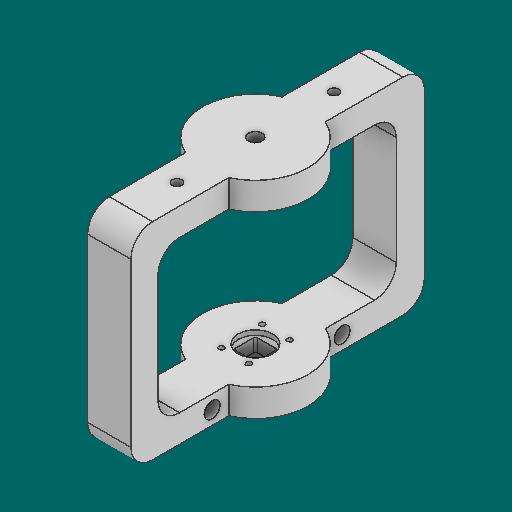
# Autodesk Inventor part: Linear_Odom
Saved by Autodesk Inventor 2025.2 (Build 292293000, 293)
## iProperties
Created: 2024-11-26
Part Number: Linear_Odom
Material: Generic
Document SubType Name: Modeling
Designer: AtuStem
Density: 1 g/cm^3
Appearance: Default
Author: AtuStem
Autodesk Inventor part; units mm, degrees
ref_plane "YZ Plane" through (0, 0, 0) normal (1, 0, 0) x (0, 1, 0)
ref_plane "XZ Plane" through (0, 0, 0) normal (0, 1, 0) x (-1, 0, 0)
ref_plane "XY Plane" through (0, 0, 0) normal (0, 0, 1) x (1, 0, 0)
sketch "Sketch1" plane through (0, 0, 0) normal (0, 1, 0) x (-1, 0, 0)
  line L0 (-6.75, -8.275) -> (-6.75, 8.275)
  line L1 (-6.75, -8.275) -> (6.75, -8.275)
  line L2 (6.75, -8.275) -> (6.75, 8.275)
  line L3 (6.75, 8.275) -> (-6.75, 8.275)
  circle A0 centre (4, 6) radius 0.8
  circle A1 centre (4, -6) radius 0.8
  circle A2 centre (-4, 6) radius 0.8
  circle A3 centre (-4, -6) radius 0.8
  line L4 (-5.98, -14.3) -> (-3.115, -23.927)
  arc A4 (-3.115, -23.927) -> (3.115, -23.927) centre (0, -23) ccw
  line L5 (3.115, -23.927) -> (5.98, -14.3)
  arc A5 (5.98, -14.3) -> (14.8963, -4.2836) centre (0, 0) ccw
  arc A6 (14.8963, 4.2836) -> (5.98, 14.3) centre (0, 0) ccw
  line L6 (5.98, 14.3) -> (3.115, 23.927)
  arc A7 (3.115, 23.927) -> (-3.115, 23.927) centre (0, 23) ccw
  line L7 (-3.115, 23.927) -> (-5.98, 14.3)
  circle A8 centre (0, -23.0125) radius 1.435
  circle A9 centre (0, 23.0125) radius 1.435
  circle A10 centre (0, 0) radius 15.5
  line L8 (0, 0) -> (0, 34.925)
  line L9 (0, 0) -> (0, -34.925)
  line L10 (0, -34.925) -> (0, -43.18)
  line L11 (0, 34.925) -> (0, 43.18)
  line L12 (0, -43.18) -> (-6.35, -43.18)
  line L13 (0, -43.18) -> (6.35, -43.18)
  line L14 (-6.35, -43.18) -> (6.35, -43.18)
  line L15 (6.35, -43.18) -> (6.35, -34.925)
  line L16 (6.35, -34.925) -> (-6.35, -34.925)
  line L17 (-6.35, -34.925) -> (-6.35, -43.18)
  line L18 (-6.35, 34.925) -> (6.35, 34.925)
  line L19 (6.35, 34.925) -> (6.35, 42.8439)
  line L20 (6.35, 42.8439) -> (-6.35, 42.8439)
  line L21 (-6.35, 42.8439) -> (-6.35, 34.925)
  line L22 (-6.35, -34.925) -> (-6.35, -14.1396)
  line L23 (-6.35, -14.1396) -> (-6.35, -13.0566)
  line L24 (-6.35, 14.1396) -> (-6.35, 34.925)
  line L25 (6.35, -34.925) -> (6.35, -14.1396)
  line L26 (6.35, 14.1396) -> (6.35, 34.925)
  point P0 (0, 0)
  point P1 (0, 0)
  point P2 (0, 0)
  point P3 (14.8963, -4.2836)
  point P4 (14.8963, 4.2836)
  dimension "d11" = 34.925
  dimension "d12" = 34.925
  dimension "d13" = 8.255
  dimension "d14" = 8.255
  dimension "d15" = 6.35
  dimension "d16" = 6.35
  constraints: 54 end point, 12 point on circle, 11 centre point, 7 vertical, 4 horizontal, 4 parallel, 4 perpendicular, 1 coincident, 1 point on line
  measures "d11" distance of L8.start L8.end
  measures "d12" distance of L8.start L9.end
  measures "d13" distance of L9.end L10.end
  measures "d14" distance of L8.end L11.end
  measures "d15" distance of L10.end L12.end
  measures "d16" distance of L10.end L13.end
extrude "Extrusion1" add sketch "Sketch1" along normal blind 8.001 contours L0 L3 L8 L9 L1 | L9 L8 L3 L2 L1
sketch "Sketch2" plane through (0, 8.001, 0) normal (0, 1, 0) x (1, 0, 0)
  circle A0 centre (0, 0) radius 5.08
  dimension "d4" = 10.16
  constraints: 1 centre point, 1 coincident
  measures "d4" diameter of A0
extrude "Extrusion2" cut sketch "Sketch2" against normal blind 1.397
sketch "Sketch3" plane through (0, 6.604, 0) normal (0, 1, 0) x (1, 0, 0)
  line L0 (-3.2283, 2.5775) -> (-3.2283, -2.5775)
  arc A0 (-3.2283, -2.5775) -> (-2.5775, -3.2283) centre (-2.5775, -2.5775) ccw
  line L1 (-2.5775, -3.2283) -> (2.5775, -3.2283)
  arc A1 (2.5775, -3.2283) -> (3.2283, -2.5775) centre (2.5775, -2.5775) ccw
  line L2 (3.2283, -2.5775) -> (3.2283, 2.5775)
  arc A2 (3.2283, 2.5775) -> (2.5775, 3.2283) centre (2.5775, 2.5775) ccw
  line L3 (2.5775, 3.2283) -> (-2.5775, 3.2283)
  arc A3 (-2.5775, 3.2283) -> (-3.2283, 2.5775) centre (-2.5775, 2.5775) ccw
  circle A4 centre (0, 0) radius 2.0828
  constraints: 8 end point, 8 point on circle, 5 centre point
extrude "Extrusion3" cut sketch "Sketch3" against normal blind 3.81 contours A3 L3 A2 L2 A1 L1 A0 L0 | A4
extrude "Extrusion4" add sketch "Sketch1" along normal up to surface (8.001 mm away) contours L1 L9 A10 L8 L3 L0 | L1 L2 L3 L8 A10 A6 A5 L9 | L9 A8 A4 L4 A10 | A10 L5 A4 L9 A8 | L8 A9 A7 L6 A10 | A10 L7 A7 L8 A9
extrude "Extrusion5" add sketch "Sketch1" along normal up to surface (8.001 mm away) contours L4 A4 L9 L16 L22 A10 | A5 L25 L16 L9 A4 L5 | L6 A7 L8 L18 L26 A6 | A10 L24 L18 L8 A7 L7
extrude "Extrusion6" add sketch "Sketch1" along normal up to surface (8.001 mm away) contours L16 L10 L12 L17 | L15 L13 L10 L16 | L18 L11 L20 L19 | L21 L20 L11 L18
sketch "Sketch5" plane through (0, 8.001, 0) normal (0, 1, 0) x (1, 0, 0)
  arc A0 (6.35, -14.1396) -> (6.35, 14.1396) centre (0, 0) ccw projected
  line L0 (6.35, 43.18) -> (6.35, 14.1396) projected
  line L1 (-6.35, 43.18) -> (6.35, 43.18) projected
  line L2 (-6.35, 14.1396) -> (-6.35, 43.18) projected
  arc A1 (-6.35, 14.1396) -> (-6.35, -14.1396) centre (0, 0) ccw projected
  line L3 (-6.35, -42.8439) -> (-6.35, -14.1396) projected
  line L4 (6.35, -42.8439) -> (-6.35, -42.8439) projected
  line L5 (6.35, -14.1396) -> (6.35, -42.8439) projected
  circle A2 centre (0, 23.0125) radius 1.435 projected
  circle A3 centre (0, -23.0125) radius 1.435 projected
  circle A4 centre (0, 0) radius 5.08 projected
  circle A5 centre (-4, -6) radius 0.8 projected
  circle A6 centre (-4, 6) radius 0.8 projected
  circle A7 centre (4, -6) radius 0.8 projected
  circle A8 centre (4, 6) radius 0.8 projected
  line L6 (-6.35, 34.925) -> (6.35, 34.925) projected
  line L7 (6.35, -34.925) -> (-6.35, -34.925) projected
extrude "Extrusion7" add sketch "Sketch5" along normal blind 44.45 contours L5 L4 L3 L7 | L6 L2 L1 L0
fillet "Fillet1" radius 6.35 2 edges at (0, 8.001, -34.925) (0, 8.001, 34.925)
sketch "Sketch6" plane through (0, 52.451, 0) normal (0, 1, 0) x (1, 0, 0)
  line L0 (-6.35, 34.925) -> (6.35, 34.925) projected
  line L1 (-6.35, 43.18) -> (-6.35, 34.925) projected
  line L2 (-6.35, 34.925) -> (6.35, 34.925) projected
  line L3 (6.35, 34.925) -> (6.35, 43.18) projected
  line L4 (6.35, 43.18) -> (-6.35, 43.18) projected
  line L5 (6.35, -42.8439) -> (6.35, -34.925) projected
  line L6 (6.35, -34.925) -> (-6.35, -34.925) projected
  line L7 (-6.35, -34.925) -> (-6.35, -42.8439) projected
  line L8 (-6.35, -42.8439) -> (6.35, -42.8439) projected
  point P0 (0, 0)
extrude "Extrusion8" add sketch "Sketch6" along normal blind 8.001
sketch "Sketch7" plane through (-6.35, 0, 42.8439) normal (0, 0, 1) x (1, 0, 0)
  line L0 (0, 0) -> (0, 60.452) projected
  line L1 (0, 0) -> (12.7, 0) projected
  line L2 (12.7, 0) -> (12.7, 60.452) projected
  line L3 (0, 60.452) -> (12.7, 60.452) projected
  line L4 (0, 60.452) -> (0, 52.451)
  line L5 (0, 52.451) -> (12.7, 52.451)
  point P0 (6.35, 0)
  dimension "d26" = 8.001
  constraints: 4 end point, 2 point on line, 1 perpendicular
  measures "d26" distance of L0.end L4.end
extrude "Extrusion9" add sketch "Sketch7" against normal up to surface (77.7689 mm away) contours L0 L3 L2 L5
fillet "Fillet2" radius 6.35 4 edges at (0, 0, 42.8439) (0, 60.452, 42.8439) (0, 60.452, -43.18) (0, 0, -43.18)
fillet "Fillet3" radius 6.35 2 edges at (0, 52.451, -34.925) (0, 52.451, 34.925)
sketch "Sketch9" plane through (-6.35, 52.451, 28.575) normal (0, -1, 0) x (1, 0, 0)
  circle A0 centre (6.35, -28.575) radius 2.032
  circle A1 centre (6.35, -28.575) radius 5.08
  dimension "d31" = 4.064
  dimension "d32" = 10.16
  constraints: 2 centre point, 2 coincident
  measures "d31" diameter of A0
  measures "d32" diameter of A1
extrude "Extrusion10" cut sketch "Sketch9" against normal blind 1.397 contours A0 | A1
sketch "Sketch10" plane through (0, 8.001, 0) normal (0, 1, 0) x (1, 0, 0)
  line L0 (-2.5775, 3.2283) -> (2.5775, 3.2283) projected
  arc A0 (-2.5775, 3.2283) -> (-3.2283, 2.5775) centre (-2.5775, 2.5775) ccw projected
  line L1 (-3.2283, -2.5775) -> (-3.2283, 2.5775) projected
  arc A1 (-3.2283, -2.5775) -> (-2.5775, -3.2283) centre (-2.5775, -2.5775) ccw projected
  line L2 (2.5775, -3.2283) -> (-2.5775, -3.2283) projected
  arc A2 (2.5775, -3.2283) -> (3.2283, -2.5775) centre (2.5775, -2.5775) ccw projected
  line L3 (3.2283, 2.5775) -> (3.2283, -2.5775) projected
  arc A3 (3.2283, 2.5775) -> (2.5775, 3.2283) centre (2.5775, 2.5775) ccw projected
  point P0 (0, 0)
sketch "Sketch11" plane through (0, 53.848, 0) normal (0, -1, 0) x (1, 0, 0)
  line L0 (-2.5775, 3.2283) -> (2.5775, 3.2283)
  arc A0 (-2.5775, 3.2283) -> (-3.2283, 2.5775) centre (-2.5775, 2.5775) ccw
  line L1 (-3.2283, -2.5775) -> (-3.2283, 2.5775)
  arc A1 (-3.2283, -2.5775) -> (-2.5775, -3.2283) centre (-2.5775, -2.5775) ccw
  line L2 (2.5775, -3.2283) -> (-2.5775, -3.2283)
  arc A2 (2.5775, -3.2283) -> (3.2283, -2.5775) centre (2.5775, -2.5775) ccw
  line L3 (3.2283, 2.5775) -> (3.2283, -2.5775)
  arc A3 (3.2283, 2.5775) -> (2.5775, 3.2283) centre (2.5775, 2.5775) ccw
  point P0 (0, 0)
  point P1 (0, 0)
  constraints: 8 end point, 8 point on circle, 4 centre point
extrude "Extrusion11" cut sketch "Sketch11" against normal blind 3.81
sketch "Sketch12" plane through (0, 60.452, 0) normal (0, 1, 0) x (1, 0, 0)
  circle A0 centre (0, 0) radius 2.032
  dimension "d37" = 4.064
  constraints: 1 centre point, 1 coincident
  measures "d37" diameter of A0
extrude "Extrusion12" cut sketch "Sketch12" against normal blind 12.7
extrude "Extrusion14" cut sketch "Sketch1" along normal through all both and the other way through all contours L9 A8 | A8 L9 | L8 A9 | A9 L8
sketch "Sketch14" plane through (0, 60.452, 0) normal (0, 1, 0) x (1, 0, 0)
  arc A0 (-6.35, 14.1396) -> (-6.35, -14.1396) centre (0, 0) ccw projected
  line L0 (6.35, -28.575) -> (-6.35, -28.575) projected
  line L1 (6.35, -14.1396) -> (6.35, -28.575) projected
  arc A1 (6.35, -14.1396) -> (6.35, 14.1396) centre (0, 0) ccw projected
  line L2 (6.35, 28.575) -> (6.35, 14.1396) projected
  line L3 (-6.35, 28.575) -> (6.35, 28.575) projected
  line L4 (-6.35, 14.1396) -> (-6.35, 28.575) projected
  arc A2 (-6.35, 14.1396) -> (-6.35, -14.1396) centre (0, 0) ccw projected
  line L5 (-6.35, -28.575) -> (-6.35, -14.1396) projected
  circle A3 centre (4, 6) radius 0.8 projected
  circle A4 centre (4, -6) radius 0.8 projected
  circle A5 centre (-4, 6) radius 0.8 projected
  circle A6 centre (-4, -6) radius 0.8 projected
  circle A7 centre (0, 0) radius 5.08 projected
  circle A8 centre (0, -23.0125) radius 1.435 projected
  circle A9 centre (0, 23.0125) radius 1.435 projected
  point P0 (-6.35, -14.1396)
  point P1 (-6.35, 14.1396)
extrude "Extrusion15" add sketch "Sketch14" against normal up to surface (8.001 mm away)
extrude "Extrusion16" add sketch "Sketch1" along normal up to surface (8.001 mm away) contours L9 A8 | A8 L9 | L8 A9 | A9 L8
sketch "Sketch15" plane through (-6.35, 0, 14.1396) normal (-1, 0, 0) x (0, 0, 1)
  line L0 (-14.1396, 0) -> (-45.8896, 0)
  line L1 (0, 0) -> (-28.2791, 0) projected
  line L2 (-14.1396, 0) -> (17.6104, 0)
  line L3 (-28.2791, 8.001) -> (0, 8.001) projected
  line L4 (0, 0) -> (0, 8.001) projected
  line L5 (0, 8.001) -> (-28.2791, 8.001) projected
  line L6 (-28.2791, 8.001) -> (-28.2791, 0) projected
  line L7 (-28.2791, 0) -> (0, 0) projected
  line L8 (-14.1396, 0) -> (-14.1396, 8.001)
  line L9 (-14.1396, 4.0005) -> (17.6104, 4.0005)
  line L10 (-14.1396, 4.0005) -> (-45.8896, 4.0005)
  circle A0 centre (-45.8896, 4.0005) radius 2.3241
  circle A1 centre (17.6104, 4.0005) radius 2.3241
  line L11 (17.6104, 4.0005) -> (11.2604, 4.0005)
  line L12 (-45.8896, 4.0005) -> (-39.5396, 4.0005)
  line L13 (11.2604, 4.0005) -> (4.9104, 4.0005)
  line L14 (-39.5396, 4.0005) -> (-33.1896, 4.0005)
  circle A2 centre (4.9104, 4.0005) radius 2.3241
  circle A3 centre (-33.1896, 4.0005) radius 2.3241
  line L15 (-57.3196, 6.35) -> (-57.3196, 54.102) projected
  line L16 (-57.3196, 30.226) -> (28.7043, 30.226)
  line L17 (28.7043, 6.35) -> (28.7043, 54.102) projected
  line L18 (-14.1396, 60.452) -> (-45.8896, 60.452)
  line L19 (0, 60.452) -> (-28.2791, 60.452)
  line L20 (-14.1396, 60.452) -> (17.6104, 60.452)
  line L21 (-28.2791, 52.451) -> (0, 52.451)
  line L22 (0, 60.452) -> (0, 52.451)
  line L23 (0, 52.451) -> (-28.2791, 52.451)
  line L24 (-28.2791, 52.451) -> (-28.2791, 60.452)
  line L25 (-28.2791, 60.452) -> (0, 60.452)
  line L26 (-14.1396, 60.452) -> (-14.1396, 52.451)
  line L27 (-14.1396, 56.4515) -> (17.6104, 56.4515)
  line L28 (-14.1396, 56.4515) -> (-45.8896, 56.4515)
  circle A4 centre (-45.8896, 56.4515) radius 2.3241
  circle A5 centre (17.6104, 56.4515) radius 2.3241
  line L29 (17.6104, 56.4515) -> (11.2604, 56.4515)
  line L30 (-45.8896, 56.4515) -> (-39.5396, 56.4515)
  line L31 (11.2604, 56.4515) -> (4.9104, 56.4515)
  line L32 (-39.5396, 56.4515) -> (-33.1896, 56.4515)
  circle A6 centre (4.9104, 56.4515) radius 2.3241
  circle A7 centre (-33.1896, 56.4515) radius 2.3241
  dimension "d52" = 31.75
  dimension "d53" = 31.75
  dimension "d54" = 4.6482
  dimension "d55" = 4.6482
  dimension "d58" = 6.35
  dimension "d59" = 6.35
  dimension "d60" = 6.35
  dimension "d61" = 6.35
  constraints: 50 end point, 23 symmetric about line, 10 point on line, 8 centre point, 8 coincident, 4 midpoint, 2 horizontal, 1 collinear, 4 other
  measures "d52" distance of L0.start L0.end
  measures "d53" distance of L0.start L2.end
  measures "d54" diameter of A0
  measures "d55" diameter of A1
  measures "d58" distance of L11.start L11.end
  measures "d59" distance of L12.start L12.end
  measures "d60" distance of L11.end L13.end
  measures "d61" distance of L12.end L14.end
extrude "Extrusion18" cut sketch "Sketch15" along normal through all both and the other way through all contours L9 A2 | L9 A2 | A3 L10 | L10 A3
body "Solid1"
